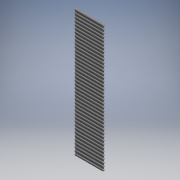
# Autodesk Inventor part: IDSD-20-S-2_ce
Saved by Autodesk Inventor 2017.3 (Build 213256000, 256)
## iProperties
Part Number: IDSD-20-S-2_ce
Material: Generic
Catalog Web Link: www.cadenas.de
Description: IDSS, IDSD Series - End Cable-.100" Slim Body, IDC Ribbon Cable Assembly, Socket
Vendor: SAMTEC
Document SubType Name: Modeling
Designer: partserver
Manufacturer: SAMTEC
Mass: 0.320706 g
Surface Area: 14.4181 cm^2
Volume: 0.320706 cm^3
Density: 1 g/cm^3
Appearance: PSOLRGB-175-175-175
Category: PARTsolutions
Company: SAMTEC
Title: IDSD-20-S-2_ce
Author: Cadenas PARTsolutions
Comments: .100" Slim Body, IDC Ribbon Cable Assembly, Socket
PSOL_IDENT_0: {$CADENAS_DATA\23d-libs\samtec\modelling\idsd\parts\idsd_end_cable.prj},269 {VTYP=3D},{NB=IDSD-20-S-
PSOL_IDENT_1: 2_ce},{LINA=IDSD-20-S-2_ce},{NN=IDSS, IDSD Series - End Cable},{DATE=12.08.2019 09:04:52},{GEOMDATE=
PSOL_IDENT_2: 25.07.2016 08:23:57},{VERSION=},{LINEID=30},{WBVAR=POS,EA,AL,PLOPT,WCC,RWOPT,POLOPT,DOPT,DOPTCT,ROPT
PSOL_IDENT_3: ,MOPT,OOPT,BOOPT,STOPT},{WBNUMERIC=AL,DOPT}  {NB=IDSD-20-S-2_ce},{LINA=IDSD-20-S-2_ce},{KT=DUMMY},{P
PSOL_IDENT_4: N=IDSD-20-S-2},{SERIES=IDSD},{POS=20},{POSNO=20},{EA=S},{EANO=1},{AL=2.00},{PLOPT=},{PLOPTDASH=},{WC
PSOL_IDENT_5: C=},{WCCALG= '','Standard Color Coded Cable','G','-G - Gray Cable' },{WCCDASH=},{RWOPT=},{RWOPTDASH=
PSOL_IDENT_6: },{POLOPT=Not Selected},{POLOPTALG='01','02','03','04','05','06','07','08','09','10','11','12','13','
PSOL_IDENT_7: 14','15','16','17','18','19','20','21','22','23','24','25','26','27','28','29','30','31','32','33','
PSOL_IDENT_8: 34','35','36','37','38','39','40'},{POLOPTMAX='01','02','03','04','05','06','07','08','09','10','11'
PSOL_IDENT_9: ,'12','13','14','15','16','17','18','19','20','21','22','23','24','25','26','27','28','29','30','31'
PSOL_IDENT_10: ,'32','33','34','35','36','37','38','39','40','41','42','43','44','45','46','47','48','49','50','51'
PSOL_IDENT_11: ,'52','53','54','55','56','57','58','59','60','61','62','63','64','65','66','67','68','69','70','71'
PSOL_IDENT_12: ,'72'},{POLOPTCTF=40},{POLOPTPN=},{POLOPTNO=0},{ROWNO=2},{DOPT=0},{DOPTCT=},{DOPTCTALG= '','Not Avai
PSOL_IDENT_13: lable' },{DOPTPN=},{ROPT=},{ROPTALG= '','Not Selected','R','-R - Reversed' },{ROPTDASH=},{MOPT=},{MO
PSOL_IDENT_14: PTALG= '','Not Available' },{MOPTDASH=},{OOPT=},{OOPTALG= '','Not Available' },{OOPTDASH=},{BOOPT=No
PSOL_IDENT_15: t Selected},{BOOPTALG='01','02','03','04','05','06','07','08','09','10','11','12','13','14','15','16'
PSOL_IDENT_16: ,'17','18','19','20','21','22','23','24','25','26','27','28','29','30','31','32','33','34','35','36'
PSOL_IDENT_17: ,'37','38','39'},{BOOPTMAX='01','02','03','04','05','06','07','08','09','10','11','12','13','14','15'
PSOL_IDENT_18: ,'16','17','18','19','20','21','22','23','24','25','26','27','28','29','30','31','32','33','34','35'
PSOL_IDENT_19: ,'36','37','38','39','40','41','42','43','44','45','46','47','48','49','50','51','52','53','54','55'
PSOL_IDENT_20: ,'56','57','58','59','60','61','62','63','64','65','66','67','68','69','70','71','72'},{BOOPTCTF=40}
PSOL_IDENT_21: ,{BOOPTPN=},{BOOPTNO=0},{STOPT=},{STOPTALG= '','Not Selected','ST8','-ST8 - 1/8\" (3.18)','ST4','-ST
PSOL_IDENT_22: 4 - 1/4\" (6.35)','ST2','-ST2 - 1/2\" (12.7)','ST3','-ST3 - 3/8\" (9.53)' },{STOPTDASH=},{L=0.250},{
PSOL_IDENT_23: B=0.2}
NB: IDSD-20-S-2_ce
NN: IDSS, IDSD Series - End Cable
NT: .100" Slim Body, IDC Ribbon Cable Assembly, Socket
NBSYN: $PN._ce
LINA: IDSD-20-S-2_ce
CATALOG: Samtec
PN: IDSD-20-S-2
SERIES: IDSD
POS: -20
EA: -S - Single End
AL: 2
PLOPT: Standard - Selective Gold
WCC: Standard Color Coded Cable
RWOPT: Not Selected
POLOPT: Not Selected
DOPT: 0
DOPTCT: Not Available
ROPT: Not Selected
MOPT: Not Available
OOPT: Not Available
BOOPT: Not Selected
STOPT: Not Selected
B: 0.2
SUPPLIER: SAMTEC
ARTICLENO: IDSD-20-S-2_ce
BOMINFO: IDSD-20-S-2_ce
CREATOR: CADENAS GmbH
Autodesk Inventor part; units mm, degrees
sketch "Sketch_1" plane through (-2.0955, 0, 0) normal (1, 0, 0) x (0, 0, -1)
  arc A0 (-24.339, 0.127) -> (-24.339, -0.127) centre (-24.765, 0) ccw
  line L0 (-24.339, -0.127) -> (-23.921, -0.127)
  arc A1 (-23.921, -0.127) -> (-23.069, -0.127) centre (-23.495, 0) ccw
  line L1 (-23.069, -0.127) -> (-22.651, -0.127)
  arc A2 (-22.651, -0.127) -> (-21.799, -0.127) centre (-22.225, 0) ccw
  line L2 (-21.799, -0.127) -> (-21.381, -0.127)
  arc A3 (-21.381, -0.127) -> (-20.529, -0.127) centre (-20.955, 0) ccw
  line L3 (-20.529, -0.127) -> (-20.111, -0.127)
  arc A4 (-20.111, -0.127) -> (-19.259, -0.127) centre (-19.685, 0) ccw
  line L4 (-19.259, -0.127) -> (-18.841, -0.127)
  arc A5 (-18.841, -0.127) -> (-17.989, -0.127) centre (-18.415, 0) ccw
  line L5 (-17.989, -0.127) -> (-17.571, -0.127)
  arc A6 (-17.571, -0.127) -> (-16.719, -0.127) centre (-17.145, 0) ccw
  line L6 (-16.719, -0.127) -> (-16.301, -0.127)
  arc A7 (-16.301, -0.127) -> (-15.449, -0.127) centre (-15.875, 0) ccw
  line L7 (-15.449, -0.127) -> (-15.031, -0.127)
  arc A8 (-15.031, -0.127) -> (-14.179, -0.127) centre (-14.605, 0) ccw
  line L8 (-14.179, -0.127) -> (-13.761, -0.127)
  arc A9 (-13.761, -0.127) -> (-12.909, -0.127) centre (-13.335, 0) ccw
  line L9 (-12.909, -0.127) -> (-12.491, -0.127)
  arc A10 (-12.491, -0.127) -> (-11.639, -0.127) centre (-12.065, 0) ccw
  line L10 (-11.639, -0.127) -> (-11.221, -0.127)
  arc A11 (-11.221, -0.127) -> (-10.369, -0.127) centre (-10.795, 0) ccw
  line L11 (-10.369, -0.127) -> (-9.951, -0.127)
  arc A12 (-9.951, -0.127) -> (-9.099, -0.127) centre (-9.525, 0) ccw
  line L12 (-9.099, -0.127) -> (-8.681, -0.127)
  arc A13 (-8.681, -0.127) -> (-7.829, -0.127) centre (-8.255, 0) ccw
  line L13 (-7.829, -0.127) -> (-7.411, -0.127)
  arc A14 (-7.411, -0.127) -> (-6.559, -0.127) centre (-6.985, 0) ccw
  line L14 (-6.559, -0.127) -> (-6.141, -0.127)
  arc A15 (-6.141, -0.127) -> (-5.289, -0.127) centre (-5.715, 0) ccw
  line L15 (-5.289, -0.127) -> (-4.871, -0.127)
  arc A16 (-4.871, -0.127) -> (-4.019, -0.127) centre (-4.445, 0) ccw
  line L16 (-4.019, -0.127) -> (-3.601, -0.127)
  arc A17 (-3.601, -0.127) -> (-2.749, -0.127) centre (-3.175, 0) ccw
  line L17 (-2.749, -0.127) -> (-2.331, -0.127)
  arc A18 (-2.331, -0.127) -> (-1.479, -0.127) centre (-1.905, 0) ccw
  line L18 (-1.479, -0.127) -> (-1.061, -0.127)
  arc A19 (-1.061, -0.127) -> (-0.209, -0.127) centre (-0.635, 0) ccw
  line L19 (-0.209, -0.127) -> (0.209, -0.127)
  arc A20 (0.209, -0.127) -> (1.061, -0.127) centre (0.635, 0) ccw
  line L20 (1.061, -0.127) -> (1.479, -0.127)
  arc A21 (1.479, -0.127) -> (2.331, -0.127) centre (1.905, 0) ccw
  line L21 (2.331, -0.127) -> (2.749, -0.127)
  arc A22 (2.749, -0.127) -> (3.601, -0.127) centre (3.175, 0) ccw
  line L22 (3.601, -0.127) -> (4.019, -0.127)
  arc A23 (4.019, -0.127) -> (4.871, -0.127) centre (4.445, 0) ccw
  line L23 (4.871, -0.127) -> (5.289, -0.127)
  arc A24 (5.289, -0.127) -> (6.141, -0.127) centre (5.715, 0) ccw
  line L24 (6.141, -0.127) -> (6.559, -0.127)
  arc A25 (6.559, -0.127) -> (7.411, -0.127) centre (6.985, 0) ccw
  line L25 (7.411, -0.127) -> (7.829, -0.127)
  arc A26 (7.829, -0.127) -> (8.681, -0.127) centre (8.255, 0) ccw
  line L26 (8.681, -0.127) -> (9.099, -0.127)
  arc A27 (9.099, -0.127) -> (9.951, -0.127) centre (9.525, 0) ccw
  line L27 (9.951, -0.127) -> (10.369, -0.127)
  arc A28 (10.369, -0.127) -> (11.221, -0.127) centre (10.795, 0) ccw
  line L28 (11.221, -0.127) -> (11.639, -0.127)
  arc A29 (11.639, -0.127) -> (12.491, -0.127) centre (12.065, 0) ccw
  line L29 (12.491, -0.127) -> (12.909, -0.127)
  arc A30 (12.909, -0.127) -> (13.761, -0.127) centre (13.335, 0) ccw
  line L30 (13.761, -0.127) -> (14.179, -0.127)
  arc A31 (14.179, -0.127) -> (15.031, -0.127) centre (14.605, 0) ccw
  line L31 (15.031, -0.127) -> (15.449, -0.127)
  arc A32 (15.449, -0.127) -> (16.301, -0.127) centre (15.875, 0) ccw
  line L32 (16.301, -0.127) -> (16.719, -0.127)
  arc A33 (16.719, -0.127) -> (17.571, -0.127) centre (17.145, 0) ccw
  line L33 (17.571, -0.127) -> (17.989, -0.127)
  arc A34 (17.989, -0.127) -> (18.841, -0.127) centre (18.415, 0) ccw
  line L34 (18.841, -0.127) -> (19.259, -0.127)
  arc A35 (19.259, -0.127) -> (20.111, -0.127) centre (19.685, 0) ccw
  line L35 (20.111, -0.127) -> (20.529, -0.127)
  arc A36 (20.529, -0.127) -> (21.381, -0.127) centre (20.955, 0) ccw
  line L36 (21.381, -0.127) -> (21.799, -0.127)
  arc A37 (21.799, -0.127) -> (22.651, -0.127) centre (22.225, 0) ccw
  line L37 (22.651, -0.127) -> (23.069, -0.127)
  arc A38 (23.069, -0.127) -> (23.921, -0.127) centre (23.495, 0) ccw
  line L38 (23.921, -0.127) -> (24.339, -0.127)
  arc A39 (24.339, -0.127) -> (24.339, 0.127) centre (24.765, 0) ccw
  line L39 (24.339, 0.127) -> (23.921, 0.127)
  arc A40 (23.921, 0.127) -> (23.069, 0.127) centre (23.495, 0) ccw
  line L40 (23.069, 0.127) -> (22.651, 0.127)
  arc A41 (22.651, 0.127) -> (21.799, 0.127) centre (22.225, 0) ccw
  line L41 (21.799, 0.127) -> (21.381, 0.127)
  arc A42 (21.381, 0.127) -> (20.529, 0.127) centre (20.955, 0) ccw
  line L42 (20.529, 0.127) -> (20.111, 0.127)
  arc A43 (20.111, 0.127) -> (19.259, 0.127) centre (19.685, 0) ccw
  line L43 (19.259, 0.127) -> (18.841, 0.127)
  arc A44 (18.841, 0.127) -> (17.989, 0.127) centre (18.415, 0) ccw
  line L44 (17.989, 0.127) -> (17.571, 0.127)
  arc A45 (17.571, 0.127) -> (16.719, 0.127) centre (17.145, 0) ccw
  line L45 (16.719, 0.127) -> (16.301, 0.127)
  arc A46 (16.301, 0.127) -> (15.449, 0.127) centre (15.875, 0) ccw
  line L46 (15.449, 0.127) -> (15.031, 0.127)
  arc A47 (15.031, 0.127) -> (14.179, 0.127) centre (14.605, 0) ccw
  line L47 (14.179, 0.127) -> (13.761, 0.127)
  arc A48 (13.761, 0.127) -> (12.909, 0.127) centre (13.335, 0) ccw
  line L48 (12.909, 0.127) -> (12.491, 0.127)
  arc A49 (12.491, 0.127) -> (11.639, 0.127) centre (12.065, 0) ccw
  line L49 (11.639, 0.127) -> (11.221, 0.127)
  arc A50 (11.221, 0.127) -> (10.369, 0.127) centre (10.795, 0) ccw
  line L50 (10.369, 0.127) -> (9.951, 0.127)
  arc A51 (9.951, 0.127) -> (9.099, 0.127) centre (9.525, 0) ccw
  line L51 (9.099, 0.127) -> (8.681, 0.127)
  arc A52 (8.681, 0.127) -> (7.829, 0.127) centre (8.255, 0) ccw
  line L52 (7.829, 0.127) -> (7.411, 0.127)
  arc A53 (7.411, 0.127) -> (6.559, 0.127) centre (6.985, 0) ccw
  line L53 (6.559, 0.127) -> (6.141, 0.127)
  arc A54 (6.141, 0.127) -> (5.289, 0.127) centre (5.715, 0) ccw
  line L54 (5.289, 0.127) -> (4.871, 0.127)
  arc A55 (4.871, 0.127) -> (4.019, 0.127) centre (4.445, 0) ccw
  line L55 (4.019, 0.127) -> (3.601, 0.127)
  arc A56 (3.601, 0.127) -> (2.749, 0.127) centre (3.175, 0) ccw
  line L56 (2.749, 0.127) -> (2.331, 0.127)
  arc A57 (2.331, 0.127) -> (1.479, 0.127) centre (1.905, 0) ccw
  line L57 (1.479, 0.127) -> (1.061, 0.127)
  arc A58 (1.061, 0.127) -> (0.209, 0.127) centre (0.635, 0) ccw
  line L58 (0.209, 0.127) -> (-0.209, 0.127)
  arc A59 (-0.209, 0.127) -> (-1.061, 0.127) centre (-0.635, 0) ccw
  line L59 (-1.061, 0.127) -> (-1.479, 0.127)
  arc A60 (-1.479, 0.127) -> (-2.331, 0.127) centre (-1.905, 0) ccw
  line L60 (-2.331, 0.127) -> (-2.749, 0.127)
  arc A61 (-2.749, 0.127) -> (-3.601, 0.127) centre (-3.175, 0) ccw
  line L61 (-3.601, 0.127) -> (-4.019, 0.127)
  arc A62 (-4.019, 0.127) -> (-4.871, 0.127) centre (-4.445, 0) ccw
  line L62 (-4.871, 0.127) -> (-5.289, 0.127)
  arc A63 (-5.289, 0.127) -> (-6.141, 0.127) centre (-5.715, 0) ccw
  line L63 (-6.141, 0.127) -> (-6.559, 0.127)
  arc A64 (-6.559, 0.127) -> (-7.411, 0.127) centre (-6.985, 0) ccw
  line L64 (-7.411, 0.127) -> (-7.829, 0.127)
  arc A65 (-7.829, 0.127) -> (-8.681, 0.127) centre (-8.255, 0) ccw
  line L65 (-8.681, 0.127) -> (-9.099, 0.127)
  arc A66 (-9.099, 0.127) -> (-9.951, 0.127) centre (-9.525, 0) ccw
  line L66 (-9.951, 0.127) -> (-10.369, 0.127)
  arc A67 (-10.369, 0.127) -> (-11.221, 0.127) centre (-10.795, 0) ccw
  line L67 (-11.221, 0.127) -> (-11.639, 0.127)
  arc A68 (-11.639, 0.127) -> (-12.491, 0.127) centre (-12.065, 0) ccw
  line L68 (-12.491, 0.127) -> (-12.909, 0.127)
  arc A69 (-12.909, 0.127) -> (-13.761, 0.127) centre (-13.335, 0) ccw
  line L69 (-13.761, 0.127) -> (-14.179, 0.127)
  arc A70 (-14.179, 0.127) -> (-15.031, 0.127) centre (-14.605, 0) ccw
  line L70 (-15.031, 0.127) -> (-15.449, 0.127)
  arc A71 (-15.449, 0.127) -> (-16.301, 0.127) centre (-15.875, 0) ccw
  line L71 (-16.301, 0.127) -> (-16.719, 0.127)
  arc A72 (-16.719, 0.127) -> (-17.571, 0.127) centre (-17.145, 0) ccw
  line L72 (-17.571, 0.127) -> (-17.989, 0.127)
  arc A73 (-17.989, 0.127) -> (-18.841, 0.127) centre (-18.415, 0) ccw
  line L73 (-18.841, 0.127) -> (-19.259, 0.127)
  arc A74 (-19.259, 0.127) -> (-20.111, 0.127) centre (-19.685, 0) ccw
  line L74 (-20.111, 0.127) -> (-20.529, 0.127)
  arc A75 (-20.529, 0.127) -> (-21.381, 0.127) centre (-20.955, 0) ccw
  line L75 (-21.381, 0.127) -> (-21.799, 0.127)
  arc A76 (-21.799, 0.127) -> (-22.651, 0.127) centre (-22.225, 0) ccw
  line L76 (-22.651, 0.127) -> (-23.069, 0.127)
  arc A77 (-23.069, 0.127) -> (-23.921, 0.127) centre (-23.495, 0) ccw
  line L77 (-23.921, 0.127) -> (-24.339, 0.127)
  constraints: 156 end point, 156 point on circle, 78 centre point
extrude "Extrusion1" add sketch "Sketch_1" along normal blind 10.9855
sketch "Sketch_2" plane through (-2.0955, 0, 0) normal (1, 0, 0) x (0, 0, -1)
  line L0 (25.2095, 0) -> (-25.2095, 0)
  arc A0 (-24.4058, 0.127) -> (-25.146, 0) centre (-24.765, 0) ccw
  line L1 (-24.4058, 0.127) -> (-23.8542, 0.127)
  arc A1 (-23.1358, 0.127) -> (-23.8542, 0.127) centre (-23.495, 0) ccw
  line L2 (-23.1358, 0.127) -> (-22.5842, 0.127)
  arc A2 (-21.8658, 0.127) -> (-22.5842, 0.127) centre (-22.225, 0) ccw
  line L3 (-21.8658, 0.127) -> (-21.3142, 0.127)
  arc A3 (-20.5958, 0.127) -> (-21.3142, 0.127) centre (-20.955, 0) ccw
  line L4 (-20.5958, 0.127) -> (-20.0442, 0.127)
  arc A4 (-19.3258, 0.127) -> (-20.0442, 0.127) centre (-19.685, 0) ccw
  line L5 (-19.3258, 0.127) -> (-18.7742, 0.127)
  arc A5 (-18.0558, 0.127) -> (-18.7742, 0.127) centre (-18.415, 0) ccw
  line L6 (-18.0558, 0.127) -> (-17.5042, 0.127)
  arc A6 (-16.7858, 0.127) -> (-17.5042, 0.127) centre (-17.145, 0) ccw
  line L7 (-16.7858, 0.127) -> (-16.2342, 0.127)
  arc A7 (-15.5158, 0.127) -> (-16.2342, 0.127) centre (-15.875, 0) ccw
  line L8 (-15.5158, 0.127) -> (-14.9642, 0.127)
  arc A8 (-14.2458, 0.127) -> (-14.9642, 0.127) centre (-14.605, 0) ccw
  line L9 (-14.2458, 0.127) -> (-13.6942, 0.127)
  arc A9 (-12.9758, 0.127) -> (-13.6942, 0.127) centre (-13.335, 0) ccw
  line L10 (-12.9758, 0.127) -> (-12.4242, 0.127)
  arc A10 (-11.7058, 0.127) -> (-12.4242, 0.127) centre (-12.065, 0) ccw
  line L11 (-11.7058, 0.127) -> (-11.1542, 0.127)
  arc A11 (-10.4358, 0.127) -> (-11.1542, 0.127) centre (-10.795, 0) ccw
  line L12 (-10.4358, 0.127) -> (-9.8842, 0.127)
  arc A12 (-9.1658, 0.127) -> (-9.8842, 0.127) centre (-9.525, 0) ccw
  line L13 (-9.1658, 0.127) -> (-8.6142, 0.127)
  arc A13 (-7.8958, 0.127) -> (-8.6142, 0.127) centre (-8.255, 0) ccw
  line L14 (-7.8958, 0.127) -> (-7.3442, 0.127)
  arc A14 (-6.6258, 0.127) -> (-7.3442, 0.127) centre (-6.985, 0) ccw
  line L15 (-6.6258, 0.127) -> (-6.0742, 0.127)
  arc A15 (-5.3558, 0.127) -> (-6.0742, 0.127) centre (-5.715, 0) ccw
  line L16 (-5.3558, 0.127) -> (-4.8042, 0.127)
  arc A16 (-4.0858, 0.127) -> (-4.8042, 0.127) centre (-4.445, 0) ccw
  line L17 (-4.0858, 0.127) -> (-3.5342, 0.127)
  arc A17 (-2.8158, 0.127) -> (-3.5342, 0.127) centre (-3.175, 0) ccw
  line L18 (-2.8158, 0.127) -> (-2.2642, 0.127)
  arc A18 (-1.5458, 0.127) -> (-2.2642, 0.127) centre (-1.905, 0) ccw
  line L19 (-1.5458, 0.127) -> (-0.9942, 0.127)
  arc A19 (-0.2758, 0.127) -> (-0.9942, 0.127) centre (-0.635, 0) ccw
  line L20 (-0.2758, 0.127) -> (0.2758, 0.127)
  arc A20 (0.9942, 0.127) -> (0.2758, 0.127) centre (0.635, 0) ccw
  line L21 (0.9942, 0.127) -> (1.5458, 0.127)
  arc A21 (2.2642, 0.127) -> (1.5458, 0.127) centre (1.905, 0) ccw
  line L22 (2.2642, 0.127) -> (2.8158, 0.127)
  arc A22 (3.5342, 0.127) -> (2.8158, 0.127) centre (3.175, 0) ccw
  line L23 (3.5342, 0.127) -> (4.0858, 0.127)
  arc A23 (4.8042, 0.127) -> (4.0858, 0.127) centre (4.445, 0) ccw
  line L24 (4.8042, 0.127) -> (5.3558, 0.127)
  arc A24 (6.0742, 0.127) -> (5.3558, 0.127) centre (5.715, 0) ccw
  line L25 (6.0742, 0.127) -> (6.6258, 0.127)
  arc A25 (7.3442, 0.127) -> (6.6258, 0.127) centre (6.985, 0) ccw
  line L26 (7.3442, 0.127) -> (7.8958, 0.127)
  arc A26 (8.6142, 0.127) -> (7.8958, 0.127) centre (8.255, 0) ccw
  line L27 (8.6142, 0.127) -> (9.1658, 0.127)
  arc A27 (9.8842, 0.127) -> (9.1658, 0.127) centre (9.525, 0) ccw
  line L28 (9.8842, 0.127) -> (10.4358, 0.127)
  arc A28 (11.1542, 0.127) -> (10.4358, 0.127) centre (10.795, 0) ccw
  line L29 (11.1542, 0.127) -> (11.7058, 0.127)
  arc A29 (12.4242, 0.127) -> (11.7058, 0.127) centre (12.065, 0) ccw
  line L30 (12.4242, 0.127) -> (12.9758, 0.127)
  arc A30 (13.6942, 0.127) -> (12.9758, 0.127) centre (13.335, 0) ccw
  line L31 (13.6942, 0.127) -> (14.2458, 0.127)
  arc A31 (14.9642, 0.127) -> (14.2458, 0.127) centre (14.605, 0) ccw
  line L32 (14.9642, 0.127) -> (15.5158, 0.127)
  arc A32 (16.2342, 0.127) -> (15.5158, 0.127) centre (15.875, 0) ccw
  line L33 (16.2342, 0.127) -> (16.7858, 0.127)
  arc A33 (17.5042, 0.127) -> (16.7858, 0.127) centre (17.145, 0) ccw
  line L34 (17.5042, 0.127) -> (18.0558, 0.127)
  arc A34 (18.7742, 0.127) -> (18.0558, 0.127) centre (18.415, 0) ccw
  line L35 (18.7742, 0.127) -> (19.3258, 0.127)
  arc A35 (20.0442, 0.127) -> (19.3258, 0.127) centre (19.685, 0) ccw
  line L36 (20.0442, 0.127) -> (20.5958, 0.127)
  arc A36 (21.3142, 0.127) -> (20.5958, 0.127) centre (20.955, 0) ccw
  line L37 (21.3142, 0.127) -> (21.8658, 0.127)
  arc A37 (22.5842, 0.127) -> (21.8658, 0.127) centre (22.225, 0) ccw
  line L38 (22.5842, 0.127) -> (23.1358, 0.127)
  arc A38 (23.8542, 0.127) -> (23.1358, 0.127) centre (23.495, 0) ccw
  line L39 (23.8542, 0.127) -> (24.4058, 0.127)
  arc A39 (25.146, 0) -> (24.4058, 0.127) centre (24.765, 0) ccw
  line L40 (25.146, 0) -> (-25.146, 0)
  constraints: 82 end point, 80 point on circle, 40 centre point
revolve "Revolution1" add sketch "Sketch_2" angle 180 about axis through (-2.0955, 0, -25.2095) along (0, 0, 1)
ref_plane "cable_to_dummy_XY" through (0, 0, 0.1143) normal (0, 1, 0) x (1, 0, 0)
ref_plane "cable_to_dummy_YZ" through (0, 0, 0.1143) normal (1, 0, 0) x (0, 0, -1)
ref_plane "cable_to_dummy_ZX" through (0, 0, 0.1143) normal (0, 0, -1) x (0, 1, 0)
ref_plane "cable_to_lower_body_XY" through (0, 0, 0.1143) normal (0, 1, 0) x (1, 0, 0)
ref_plane "cable_to_lower_body_YZ" through (0, 0, 0.1143) normal (1, 0, 0) x (0, 0, -1)
ref_plane "cable_to_lower_body_ZX" through (0, 0, 0.1143) normal (0, 0, -1) x (0, 1, 0)
body "Solid1"
